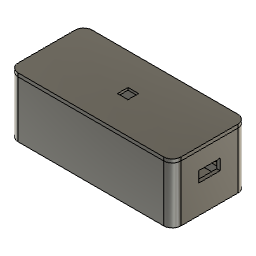
Sunrise Simulator Box v3 (Autodesk Fusion 360 design; units mm, degrees)
Autodesk Fusion 360 part; units mm, degrees
note: some values were not read from the file. Set by a fixed rule: which sketch regions a step uses.
sketch "Sketch1" plane through (0, 0, 0) normal (0, 0, 1) x (1, 0, 0)
  line L0 (0, 0) -> (91.948, 0)
  line L1 (91.948, 0) -> (91.948, 39.624)
  line L2 (91.948, 39.624) -> (0, 39.624)
  line L3 (0, 39.624) -> (0, 0)
  line L4 (-2.032, 41.656) -> (-2.032, -2.032)
  line L5 (-2.032, -2.032) -> (93.98, -2.032)
  line L6 (93.98, -2.032) -> (93.98, 41.656)
  line L7 (93.98, 41.656) -> (-2.032, 41.656)
  line L8 (1.905, 37.719) -> (1.905, 1.905)
  line L9 (1.905, 1.905) -> (90.043, 1.905)
  line L10 (90.043, 1.905) -> (90.043, 37.719)
  line L11 (90.043, 37.719) -> (1.905, 37.719)
  dimension "d1" = 91.948
  dimension "d2" = 39.624
  dimension "d3" = 2.032
  dimension "d4" = -1.905
  constraint horizontal L0
  constraint vertical L1
  constraint horizontal L2
  constraint vertical L3
  constraint coincident L0.start L3.end
  measures "d1" distance of L0.start L0.end
  measures "d2" distance of L0.start L2.end
extrude "Extrude1" add sketch "Sketch1" against normal blind 2.032 contours L0 L1 L2 L3 | L4 L5 L6 L7 | L8 L9 L10 L11 makes body 1
extrude "Extrude2" add sketch "Sketch1" along normal blind 4.445 contours L0 L1 L2 L3 bodies 1
extrude "Extrude3" add sketch "Sketch1" along normal blind 31.115 contours L4 L5 L6 L7 bodies 1
sketch "Sketch2" plane through (93.98, 0, 0) normal (1, 0, 0) x (0, 1, 0)
  line L0 (-2.032, 31.115) -> (-2.032, -2.032)
  line L1 (-2.032, -2.032) -> (41.656, -2.032)
  line L2 (41.656, -2.032) -> (41.656, 31.115)
  line L3 (41.656, 31.115) -> (-2.032, 31.115)
  line L4 (19.812, -2.032) -> (19.812, 20.955)
  line L5 (19.812, 20.955) -> (26.162, 20.955)
  line L6 (19.812, 20.955) -> (13.462, 20.955)
  line L7 (13.462, 20.955) -> (13.462, 14.605)
  line L8 (13.462, 14.605) -> (26.162, 14.605)
  line L9 (26.162, 14.605) -> (26.162, 20.955)
  dimension "d11" = 22.987
  dimension "d12" = 6.35
  dimension "d13" = 6.35
  dimension "d14" = 6.35
  constraint midpoint L1 L4.start
  constraint perpendicular L1 L4
  constraint perpendicular L4 L5
  constraint perpendicular L4 L6
  constraint perpendicular L6 L7
  constraint perpendicular L7 L8
  constraint perpendicular L5 L9
  measures "d11" distance of L4.start L4.end
  measures "d12" distance of L4.end L5.end
  measures "d13" distance of L4.end L6.end
  measures "d14" distance of L6.end L7.end
extrude "Extrude4" cut sketch "Sketch2" against normal blind 7.62 contours L4 L6 L7 L8 | L4 L5 L8 L9 bodies 1
sketch "Sketch3" plane through (-2.032, 0, 0) normal (-1, 0, 0) x (0, -1, 0)
  line L0 (-41.656, 31.115) -> (-41.656, -2.032)
  line L1 (-41.656, -2.032) -> (2.032, -2.032)
  line L2 (2.032, -2.032) -> (2.032, 31.115)
  line L3 (2.032, 31.115) -> (-41.656, 31.115)
  line L4 (-15.621, 31.0987) -> (-15.621, 24.7487)
  circle A0 centre (-15.621, 24.7487) radius 4.0005
  line L5 (-41.656, 31.115) -> (-31.496, 31.115)
  line L6 (-31.496, 31.115) -> (-31.496, 24.765)
  circle A1 centre (-31.496, 27.94) radius 3.175
  line L7 (-28.321, 27.94) -> (-28.321, 31.115)
  line L8 (-34.671, 27.94) -> (-34.671, 31.115)
  dimension "d20" = 6.35
  dimension "d21" = 8.001
  dimension "d34" = 17.653
  dimension "d35" = 10.16
  dimension "d36" = 6.35
  constraint perpendicular L3 L4
  constraint coincident L4.end A0.centre
  constraint coincident L0.start L3.end
  constraint perpendicular L0 L5
  constraint perpendicular L3 L6
  constraint midpoint L6 A1.centre
  constraint coincident L6.end A1
  constraint coincident A1 L7.start
  constraint coincident L3 L7.end
  constraint tangent A1 L7
  constraint perpendicular L3 L7
  constraint coincident A1 L8.start
  constraint coincident L3 L8.end
  measures "d20" distance of L4.start L4.end
  measures "d21" diameter of A0
  measures "d34" distance of L2 L4
  measures "d35" distance of L0.start L5.end
  measures "d36" distance of L5.end L6.end
extrude "Extrude5" cut sketch "Sketch3" against normal blind 2.54 contours L3 L5 A1 L8 | L6 A1 | L3 A1 L7 | L6 A1 | A0 bodies 1
fillet "Fillet1" radius 1.27 4 edges at (1.905, 37.719, 2.2225) (1.905, 1.905, 2.2225) (90.043, 37.719, 2.2225) (90.043, 1.905, 2.2225) on bodies 1
fillet "Fillet2" radius 3.175 4 edges at (91.948, 0, 17.78) (91.948, 39.624, 17.78) (0, 39.624, 17.78) (0, 0, 17.78) on bodies 1
fillet "Fillet3" radius 5.08 4 edges at (93.98, -2.032, 14.5415) (93.98, 41.656, 14.5415) (-2.032, -2.032, 14.5415) (-2.032, 41.656, 14.5415) on bodies 1
chamfer "Chamfer1" distance 0.635 angle 45 9 edges at (45.974, 0, 31.115) (0.9299, 0.9299, 31.115) (0, 15.748, 31.115) (0, 35.56, 31.115) (0.9299, 38.6941, 31.115) (45.974, 39.624, 31.115) (91.0181, 38.6941, 31.115) (91.948, 19.812, 31.115) (91.0181, 0.9299, 31.115) on bodies 1
fillet "Fillet5" radius 1.27 2 edges at (-1.3335, 34.671, 31.115) (-1.3335, 28.321, 31.115) on bodies 1
sketch "Sketch1 (2)" plane through (0, 0, 31.115) normal (0, 0, 1) x (-1, 0, 0) in component "Top"
  line L0 (0.635, -27.051) -> (2.032, -27.051)
  line L1 (2.032, -27.051) -> (2.032, -3.048)
  arc A0 (2.032, -3.048) -> (-3.048, 2.032) centre (-3.048, -3.048) ccw
  line L2 (-3.048, 2.032) -> (-88.9, 2.032)
  arc A1 (-88.9, 2.032) -> (-93.98, -3.048) centre (-88.9, -3.048) ccw
  line L3 (-93.98, -3.048) -> (-93.98, -36.576)
  arc A2 (-93.98, -36.576) -> (-88.9, -41.656) centre (-88.9, -36.576) ccw
  line L4 (-88.9, -41.656) -> (-3.048, -41.656)
  arc A3 (-3.048, -41.656) -> (2.032, -36.576) centre (-3.048, -36.576) ccw
  line L5 (2.032, -36.576) -> (2.032, -35.941)
  line L6 (2.032, -35.941) -> (0.635, -35.941)
  line L7 (0.635, -35.941) -> (0.635, -36.449)
  arc A4 (-3.175, -40.259) -> (0.635, -36.449) centre (-3.175, -36.449) ccw
  line L8 (-3.175, -40.259) -> (-88.773, -40.259)
  arc A5 (-92.583, -36.449) -> (-88.773, -40.259) centre (-88.773, -36.449) ccw
  line L9 (-92.583, -36.449) -> (-92.583, -3.175)
  arc A6 (-88.773, 0.635) -> (-92.583, -3.175) centre (-88.773, -3.175) ccw
  line L10 (-88.773, 0.635) -> (-3.175, 0.635)
  arc A7 (0.635, -3.175) -> (-3.175, 0.635) centre (-3.175, -3.175) ccw
  line L11 (0.635, -3.175) -> (0.635, -27.051)
  line L12 (-3.048, 4.0767) -> (-88.9, 4.0767)
  arc A8 (-88.9, 4.0767) -> (-96.0247, -3.048) centre (-88.9, -3.048) ccw
  line L13 (-96.0247, -3.048) -> (-96.0247, -36.576)
  arc A9 (-96.0247, -36.576) -> (-88.9, -43.7007) centre (-88.9, -36.576) ccw
  line L14 (-88.9, -43.7007) -> (-3.048, -43.7007)
  arc A10 (-3.048, -43.7007) -> (4.0767, -36.576) centre (-3.048, -36.576) ccw
  line L15 (4.0767, -36.576) -> (4.0767, -33.8963)
  line L16 (4.0767, -33.8963) -> (-1.4097, -33.8963)
  line L17 (-1.4097, -33.8963) -> (-1.4097, -36.449)
  arc A11 (-3.175, -38.2143) -> (-1.4097, -36.449) centre (-3.175, -36.449) ccw
  line L18 (-3.175, -38.2143) -> (-88.773, -38.2143)
  arc A12 (-90.5383, -36.449) -> (-88.773, -38.2143) centre (-88.773, -36.449) ccw
  line L19 (-90.5383, -36.449) -> (-90.5383, -3.175)
  arc A13 (-88.773, -1.4097) -> (-90.5383, -3.175) centre (-88.773, -3.175) ccw
  line L20 (-88.773, -1.4097) -> (-3.175, -1.4097)
  arc A14 (-1.4097, -3.175) -> (-3.175, -1.4097) centre (-3.175, -3.175) ccw
  line L21 (-1.4097, -3.175) -> (-1.4097, -29.0957)
  line L22 (-1.4097, -29.0957) -> (4.0767, -29.0957)
  line L23 (4.0767, -29.0957) -> (4.0767, -3.048)
  arc A15 (4.0767, -3.048) -> (-3.048, 4.0767) centre (-3.048, -3.048) ccw
  line L24 (-3.048, 2.159) -> (-88.9, 2.159)
  arc A16 (-88.9, 2.159) -> (-94.107, -3.048) centre (-88.9, -3.048) ccw
  line L25 (-94.107, -3.048) -> (-94.107, -36.576)
  arc A17 (-94.107, -36.576) -> (-88.9, -41.783) centre (-88.9, -36.576) ccw
  line L26 (-88.9, -41.783) -> (-3.048, -41.783)
  arc A18 (-3.048, -41.783) -> (2.159, -36.576) centre (-3.048, -36.576) ccw
  line L27 (2.159, -36.576) -> (2.159, -35.814)
  line L28 (2.159, -35.814) -> (0.508, -35.814)
  line L29 (0.508, -35.814) -> (0.508, -36.449)
  arc A19 (-3.175, -40.132) -> (0.508, -36.449) centre (-3.175, -36.449) ccw
  line L30 (-3.175, -40.132) -> (-88.773, -40.132)
  arc A20 (-92.456, -36.449) -> (-88.773, -40.132) centre (-88.773, -36.449) ccw
  line L31 (-92.456, -36.449) -> (-92.456, -3.175)
  arc A21 (-88.773, 0.508) -> (-92.456, -3.175) centre (-88.773, -3.175) ccw
  line L32 (-88.773, 0.508) -> (-3.175, 0.508)
  arc A22 (0.508, -3.175) -> (-3.175, 0.508) centre (-3.175, -3.175) ccw
  line L33 (0.508, -3.175) -> (0.508, -27.178)
  line L34 (0.508, -27.178) -> (2.159, -27.178)
  line L35 (2.159, -27.178) -> (2.159, -3.048)
  arc A23 (2.159, -3.048) -> (-3.048, 2.159) centre (-3.048, -3.048) ccw
  line L36 (2.032, -27.051) -> (2.032, -35.941)
  line L37 (0.635, -27.051) -> (0.635, -35.941)
  line L38 (0.635, -27.051) -> (-1.4097, -27.051)
  line L39 (0.635, -35.941) -> (-1.4097, -35.941)
  line L40 (-1.4097, -3.175) -> (4.0767, -3.175)
  dimension "d39" = 2.0447
  dimension "d40" = 0.127
  constraint coincident L0.end L1.start
  constraint coincident L5.end L6.start
  constraint coincident L0.start L11.end
  constraint coincident L6.end L7.start
  constraint coincident L21 L38.end
  constraint perpendicular L21 L38
  constraint coincident L17 L39.end
  constraint perpendicular L17 L39
  constraint coincident L23 L40.end
  constraint perpendicular L23 L40
extrude "Extrude1'" add sketch "Sketch1 (2)" along normal blind 2.032 separate body contours L0 L1 L11 L40 | L11 L33 L38 L40 | L0 L34 L36 L37 | L33 L34 L37 L38 | L7 A4 L8 A5 L9 A6 L10 A7 L29 A19 L30 A20 L31 A21 L32 A22 L39 L40 | L1 A0 L2 A1 L3 A2 L4 A3 L5 L6 L7 A4 L8 A5 L9 A6 L10 A7 L40 | L21 L22 L33 L34 L37 L38 | L22 L34 L36 L37 | L21 L33 L38 L40 | L17 A11 L18 A12 L19 A13 L20 A14 L29 A19 L30 A20 L31 A21 L32 A22 L39 L40 | L16 L17 A11 L18 A12 L19 A13 L20 A14 L21 L22 L37 | L16 L22 L36 L37 | L16 L17 L28 L29 L37 L39 | L16 L28 L36 L37 | L28 L29 L37 L39 | L6 L28 L36 L37 makes body 2 in component "Top"
extrude "Extrude2'" add sketch "Sketch1 (2)" against normal blind 3.81 contours L21 L33 L38 L40 | L17 A11 L18 A12 L19 A13 L20 A14 L29 A19 L30 A20 L31 A21 L32 A22 L39 L40 bodies 2 in component "Top"
sketch "Sketch2 (2)" plane through (0, 0, 33.147) normal (0, 0, 1) x (-1, 0, 0) in component "Top"
  arc A0 (2.032, -3.048) -> (-3.048, 2.032) centre (-3.048, -3.048) ccw
  line L0 (-3.048, 2.032) -> (-88.9, 2.032)
  arc A1 (-88.9, 2.032) -> (-93.98, -3.048) centre (-88.9, -3.048) ccw
  line L1 (-93.98, -3.048) -> (-93.98, -36.576)
  arc A2 (-93.98, -36.576) -> (-88.9, -41.656) centre (-88.9, -36.576) ccw
  line L2 (-88.9, -41.656) -> (-3.048, -41.656)
  arc A3 (-3.048, -41.656) -> (2.032, -36.576) centre (-3.048, -36.576) ccw
  line L3 (2.032, -36.576) -> (2.032, -3.048)
  line L4 (-45.974, -41.656) -> (-45.974, -19.812)
  line L5 (-49.0855, -16.7005) -> (-42.8625, -16.7005)
  line L6 (-42.8625, -16.7005) -> (-42.8625, -22.9235)
  line L7 (-42.8625, -22.9235) -> (-49.0855, -22.9235)
  line L8 (-49.0855, -22.9235) -> (-49.0855, -16.7005)
  line L9 (-49.0855, -16.7005) -> (-42.8625, -22.9235) construction
  line L10 (-42.8625, -16.7005) -> (-49.0855, -22.9235) construction
  point P0 (-45.974, -19.812)
  dimension "d45" = 6.223
  dimension "d46" = 6.223
  constraint midpoint L2 L4.start
  constraint perpendicular L2 L4
  constraint horizontal L5
  constraint perpendicular L5 L6
  constraint parallel L5 L7
  constraint parallel L6 L8
  constraint coincident L9 P0
  constraint coincident L10 P0
  constraint coincident P0 L4.end
  measures "d45" distance of L6.end L7.end
  measures "d46" distance of L5.end L6.end
extrude "Extrude3'" cut sketch "Sketch2 (2)" against normal blind 2.54 contours L5 L6 L7 L8 bodies 2 in component "Top"
extrude "Extrude4'" cut sketch "Sketch1 (2)" against normal blind 4.318 contours L21 L33 L38 L40 bodies 2 in component "Top"
fillet "Fillet1'" radius 1.27 8 edges at (1.4097, 36.195, 31.115) (1.9267, 37.6973, 31.115) (45.974, 38.2143, 31.115) (90.0213, 37.6973, 31.115) (90.5383, 19.812, 31.115) (90.0213, 1.9267, 31.115) (45.974, 1.4097, 31.115) (1.9267, 1.9267, 31.115) on bodies 2 in component "Top"
chamfer "Chamfer1'" distance 0.635 angle 45 8 edges at (-0.508, 36.195, 27.305) (0.5707, 39.0533, 27.305) (45.974, 40.132, 27.305) (91.3773, 39.0533, 27.305) (92.456, 19.812, 27.305) (91.3773, 0.5707, 27.305) (45.974, -0.508, 27.305) (0.5707, 0.5707, 27.305) on bodies 2 in component "Top"
chamfer "Chamfer2" distance 0.635 angle 45 4 edges at (42.8625, 19.812, 31.115) (45.974, 22.9235, 31.115) (49.0855, 19.812, 31.115) (45.974, 16.7005, 31.115) on bodies 2 in component "Top"
component "Top" placed x (1, 0, 0) y (0, 1, 0) z (0, 0, 1) at (0, 0, 0)
equation "d1 = 3.55 in + 0.07 in"
equation "d9 = 1.175 in + 0.05 in"
equation "d11 = 0.08 in + 0.175 in + 0.65 in"
equation "d34 = 0.86 in - 0.165 in"
